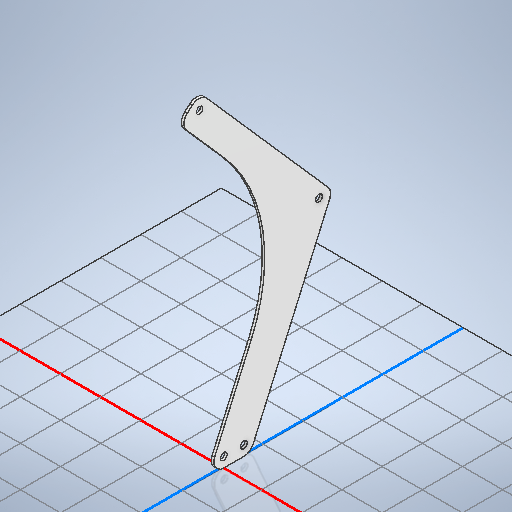
# Autodesk Inventor part: Support Gusset
Saved by Autodesk Inventor 2026 (Build 300175000, 175)
## iProperties
Created: 2025-04-06
Part Number: Support Gusset
Material: Acetal Resin, White
Document SubType Name: Modeling
Designer: avere
Density: 1.425 g/cm^3
Appearance: Smooth - White
Author: avere
Autodesk Inventor part; units mm, degrees
ref_plane "YZ Plane" through (0, 0, 0) normal (1, 0, 0) x (0, 1, 0)
ref_plane "XZ Plane" through (0, 0, 0) normal (0, 1, 0) x (-1, 0, 0)
ref_plane "XY Plane" through (0, 0, 0) normal (0, 0, 1) x (1, 0, 0)
sketch "main" plane through (0, 0, 0) normal (0, 0, 1) x (1, 0, 0)
  circle A0 centre (-11.2144, -104.2473) radius 2.1844
  circle A1 centre (1.4856, -104.2473) radius 2.1844
  circle A2 centre (48.9096, 6.9894) radius 2.1844
  circle A3 centre (-26.5889, 92.8058) radius 2.1844
  arc A4 (1.4856, -110.5973) -> (7.2979, -106.8047) centre (1.4856, -104.2473) ccw
  arc A5 (-17.0266, -101.6899) -> (-11.2144, -110.5973) centre (-11.2144, -104.2473) ccw
  line L0 (54.6905, 10.0319) -> (-22.1306, 97.3516)
  line L1 (55.7352, 3.2802) -> (7.2979, -106.8047)
  line L2 (-31.0925, 97.9248) -> (-34.2947, 95.1076)
  line L3 (-33.7837, 110.5973) -> (6.8178, 64.4472)
  line L4 (-17.0266, -101.6899) -> (6.006, -49.3432)
  line L5 (-34.8679, 86.1457) -> (-10.7088, 58.6849)
  arc A6 (-34.2947, 95.1076) -> (-34.8679, 86.1457) centre (-30.1004, 90.34) ccw
  arc A7 (-22.1306, 97.3516) -> (-31.0925, 97.9248) centre (-26.8981, 93.1573) ccw
  arc A8 (55.7352, 3.2802) -> (54.6905, 10.0319) centre (49.923, 5.8376) ccw
  arc A9 (6.006, -49.3432) -> (-10.7088, 58.6849) centre (-86.9901, -8.425) ccw
  line L6 (-11.2144, -110.5973) -> (1.4856, -110.5973)
  point P0 (16.4228, 13.0791)
  point P1 (-26.3249, 102.1192)
  point P2 (49.8339, -10.1318)
  dimension "d9" = 6.35
  dimension "d10" = 6.35
  dimension "d11" = 101.6
  measures "d9" radius of A6
  measures "d10" radius of A7
  measures "d11" radius of A9
sketch "Sketch1" plane through (0, 0, 0) normal (1, 0, 0) x (0, 1, 0)
  circle A0 centre (0, 0) radius 2.1844
  circle A1 centre (0, -12.7) radius 2.1844
  circle A2 centre (111.2367, -60.124) radius 2.1844
  circle A3 centre (197.0531, 15.3746) radius 2.1844
  arc A4 (-6.35, -12.7) -> (-2.5574, -18.5123) centre (0, -12.7) ccw
  arc A5 (2.5574, 5.8123) -> (-6.35, 0) centre (0, 0) ccw
  line L0 (114.2793, -65.9049) -> (201.599, 10.9162)
  line L1 (107.5275, -66.9496) -> (-2.5574, -18.5123)
  line L2 (202.1722, 19.8781) -> (199.3549, 23.0804)
  line L3 (214.8446, 22.5693) -> (168.6945, -18.0321)
  line L4 (2.5574, 5.8123) -> (54.9042, -17.2203)
  line L5 (190.393, 23.6536) -> (162.9322, -0.5055)
  arc A6 (199.3549, 23.0804) -> (190.393, 23.6536) centre (194.5874, 18.886) ccw
  arc A7 (201.599, 10.9162) -> (202.1722, 19.8781) centre (197.4046, 15.6838) ccw
  arc A8 (107.5275, -66.9496) -> (114.2793, -65.9049) centre (110.0849, -61.1373) ccw
  arc A9 (54.9042, -17.2203) -> (162.9322, -0.5055) centre (95.8224, 75.7757) ccw
  line L6 (-6.35, 0) -> (-6.35, -12.7)
  point P0 (0, 0)
  constraints: 1 other
extrude "Extrusion1" add sketch "Sketch1" along normal blind 1.5875
body "Solid1"
